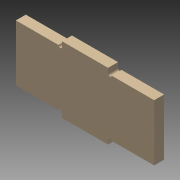
# Autodesk Inventor part: shelfSide
Saved by Autodesk Inventor 2015 SP1 (Build 190203100, 203)
## iProperties
Created: 2015-04-10
Part Number: shelfSide
Material: Generic
Document SubType Name: Modeling
Designer: Iain
Density: 1 g/cm^3
Appearance: Smooth - Off-White
Author: Iain
Autodesk Inventor part; units mm, degrees
sketch "Sketch2" plane through (0, 0, 0) normal (0, 1, 0) x (-1, 0, 0)
  line L0 (125, -60) -> (-125, -60)
  line L1 (-125, -60) -> (-125, 60)
  line L2 (-125, 60) -> (125, 60)
  line L3 (125, 60) -> (125, -60)
  point P0 (0, 0)
  point P1 (-125, 0)
  point P2 (0, -60)
  dimension "d2" = 250
  dimension "d3" = 120
  constraints: 8 end point, 2 midpoint, 2 parallel, 1 horizontal, 1 horizontal alignment, 1 perpendicular, 1 vertical alignment
  measures "d2" distance of L0.start L0.end
  measures "d3" distance of L0.end L1.end
extrude "Extrusion1" add sketch "Sketch2" along normal blind 18
sketch "Sketch3" plane through (0, 18, 0) normal (0, 1, 0) x (1, 0, 0)
  line L0 (-125, 60) -> (-41.6667, 60)
  line L1 (-41.6667, 60) -> (-41.6667, 42)
  line L2 (-41.6667, 42) -> (-125, 42)
  line L3 (-125, 42) -> (-125, 60)
  line L4 (125, 60) -> (-125, 60) projected
  line L5 (-125, 60) -> (-125, -60) projected
  line L6 (-125, -60) -> (125, -60) projected
  line L7 (125, -60) -> (125, 60) projected
  point P0 (0, 0)
  point P1 (-125, 51)
  point P2 (-125, 0)
  point P3 (-83.3333, 60)
  point P4 (0, 60)
  dimension "d6" = 83.3333
  dimension "d7" = 18
  constraints: 8 end point, 4 midpoint, 2 parallel, 1 horizontal, 1 horizontal alignment, 1 perpendicular, 1 vertical alignment
  measures "d6" distance of L0.start L0.end
  measures "d7" distance of L0.end L1.end
extrude "Extrusion2" cut sketch "Sketch3" against normal blind 18 contours L0 L1 L2 L3
ref_plane "Work Plane1" through (0, 0, 60) normal (-1, 0, 0) x (0, 0, 1)
ref_plane "Work Plane2" through (125, 0, 0) normal (0, 0, -1) x (-1, 0, 0)
mirror "Mirror1" about plane through (0, 0, 60) normal (-1, 0, 0) of "Extrusion2"
sketch "Sketch4" plane through (0, 18, 0) normal (0, 1, 0) x (1, 0, 0)
  line L0 (-41.6667, 60) -> (41.6667, 60)
  line L1 (41.6667, 60) -> (41.6667, 51)
  line L2 (41.6667, 51) -> (-41.6667, 51)
  line L3 (-41.6667, 51) -> (-41.6667, 60)
  line L4 (41.6667, 42) -> (41.6667, 60) projected
  line L5 (41.6667, 60) -> (-41.6667, 60) projected
  line L6 (-41.6667, 60) -> (-41.6667, 42) projected
  line L7 (-41.6667, 42) -> (-125, 42) projected
  line L8 (-125, 42) -> (-125, -60) projected
  line L9 (-125, -60) -> (125, -60) projected
  line L10 (125, -60) -> (125, 42) projected
  line L11 (125, 42) -> (41.6667, 42) projected
  line L12 (-41.6667, 60) -> (-41.6667, 42) projected
  point P0 (0, 0)
  point P1 (0, 60)
  point P2 (0, 60)
  point P3 (0, 51)
  point P4 (-41.6667, 51)
  point P5 (41.6667, 55.5)
  point P6 (41.6667, 51)
  point P7 (-41.6667, 55.5)
  point P8 (-41.6667, 51)
  constraints: 8 end point, 8 midpoint, 2 parallel, 2 vertical alignment, 1 coincident, 1 horizontal, 1 horizontal alignment, 1 perpendicular
extrude "Extrusion3" cut sketch "Sketch4" against normal blind 18 contours L0 L1 L2 L3
sketch "Sketch5" plane through (0, 18, 0) normal (0, 1, 0) x (1, 0, 0)
  line L0 (-41.6667, -60) -> (41.6667, -60)
  line L1 (41.6667, -60) -> (41.6667, -69)
  line L2 (41.6667, -69) -> (-41.6667, -69)
  line L3 (-41.6667, -69) -> (-41.6667, -60)
  line L4 (41.6667, 51) -> (-41.6667, 51) projected
  line L5 (-41.6667, 51) -> (-41.6667, 42) projected
  line L6 (-41.6667, 42) -> (-125, 42) projected
  line L7 (-125, 42) -> (-125, -60) projected
  line L8 (-125, -60) -> (125, -60) projected
  line L9 (125, -60) -> (125, 42) projected
  line L10 (125, 42) -> (41.6667, 42) projected
  line L11 (41.6667, 42) -> (41.6667, 51) projected
  line L12 (-125, -60) -> (125, -60) projected
  point P0 (0, 0)
  point P1 (0, -60)
  point P2 (0, -60)
  point P3 (0, -69)
  point P4 (0, -60)
  dimension "d12" = 83.3333
  dimension "d13" = 9
  constraints: 8 end point, 4 midpoint, 2 parallel, 1 coincident, 1 horizontal, 1 perpendicular, 1 vertical alignment
  measures "d12" distance of L1.end L2.end
  measures "d13" distance of L0.end L1.end
extrude "Extrusion4" add sketch "Sketch5" against normal blind 18 contours L0 L1 L2 L3
sketch "Sketch6" plane through (0, 18, 0) normal (0, 1, 0) x (1, 0, 0)
  line L0 (-41.6667, 51) -> (-41.6667, 42) projected
  line L1 (41.6667, 51) -> (41.6667, 42) projected
  point P0 (0, 0)
  point P1 (-44.8417, 42)
  point P2 (44.8417, 42)
  dimension "d16" = 3.175
  dimension "d17" = 3.175
  constraints: 2 horizontal alignment
  measures "d16" distance from line of L0 point (-44.842, 42)
  measures "d17" distance from line of L1 point (44.842, 42)
hole "Hole1" at (-44.8417, 18, -42) at (44.8417, 18, -42) direction (0, -1, 0) diameter 6.35 end through all
ref_plane "Work Plane3" through (-125, 0, 9) normal (0, 0, -1) x (-1, 0, 0)
mirror "Mirror2" about plane through (-125, 0, 9) normal (0, 0, -1) of "Hole1"
equation "\"d2\" = shelfWidth"
equation "\"d3\" = shelfHeight"
equation "\"d4\" = plyThickness"
equation "\"d6\" = 0.333333 * shelfWidth"
equation "\"d7\" = plyThickness"
equation "\"d8\" = plyThickness"
equation "\"d10\" = plyThickness"
equation "\"d12\" = 0.333333 * shelfWidth"
equation "\"d13\" = 0.5 * plyThickness"
equation "\"d14\" = plyThickness"
equation "\"d16\" = 0.5 * millDiameter"
equation "\"d17\" = 0.5 * millDiameter"
equation "\"d18\" = millDiameter"
equation "\"plyThickness\" = 18"
equation "\"legHeight\" = 702"
equation "\"millDiameter\" = 6.35"
equation "\"legTopTabHeight\" = 18"
equation "\"legTopSlotDepth\" = 49"
equation "\"shelfWidth\" = 250"
equation "\"shelfHeight\" = 120"
body "Solid1"
